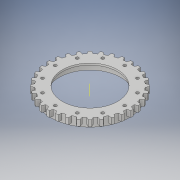
# Autodesk Inventor part: tableGear
Saved by Autodesk Inventor 2018 (Build 220112000, 112)
## iProperties
Created: 2018-04-17
Part Number: tableGear
Material: Generic
Document SubType Name: Modeling
Designer: Cole Tucker
Density: 1 g/cm^3
Appearance: Default
Author: Cole Tucker
Autodesk Inventor part; units mm, degrees
ref_plane "YZ Plane" through (0, 0, 0) normal (1, 0, 0) x (0, 1, 0)
ref_plane "XZ Plane" through (0, 0, 0) normal (0, 1, 0) x (-1, 0, 0)
ref_plane "XY Plane" through (0, 0, 0) normal (0, 0, 1) x (1, 0, 0)
sketch "Sketch1" plane through (0, 0, 0) normal (0, 1, 0) x (-1, 0, 0)
  circle A0 centre (0, 0) radius 29.21
  circle A1 centre (0, 0) radius 41.275
  dimension "d0" = 58.42
  dimension "d1" = 82.55
  constraints: 2 centre point, 2 coincident
  measures "d0" diameter of A0
  measures "d1" diameter of A1
extrude "Extrusion1" add sketch "Sketch1" along normal blind 8.89
sketch "Sketch2" plane through (0, 8.89, 0) normal (0, 1, 0) x (1, 0, 0)
  circle A0 centre (0, 0) radius 29.21 projected
  circle A1 centre (0, 0) radius 41.275 projected
  circle A2 centre (0, 0) radius 41.275 projected
  line L0 (-41.275, 0) -> (-44.45, 0)
  line L1 (-44.45, 0) -> (-44.45, 1.27)
  line L2 (-41.275, 0) -> (-40.5721, 0)
  line L3 (-40.5721, 0) -> (-40.5721, 2.54)
  line L4 (-40.5721, 2.54) -> (-44.45, 1.27)
  line L5 (-40.5721, 0) -> (-40.5721, -2.54)
  line L6 (-44.45, 0) -> (-44.45, -1.27)
  line L7 (-44.45, -1.27) -> (-40.5721, -2.54)
  dimension "d4" = 3.175
  dimension "d5" = 1.27
  dimension "d6" = 2.54
  dimension "d7" = 2.54
  dimension "d8" = 1.27
  constraints: 16 end point, 2 horizontal, 2 perpendicular, 1 horizontal alignment, 1 point on line, 1 vertical, 1 other
  measures "d4" distance of L0.start L0.end
  measures "d5" distance of L0.end L1.end
  measures "d6" distance of L2.end L3.end
  measures "d7" distance of L2.end L5.end
  measures "d8" distance of L0.end L6.end
extrude "Extrusion2" add sketch "Sketch2" against normal blind 6.35 contours L4 L3 L2 A1 | A1 L0 L1 L4 | L7 L6 L0 A1 | A1 L2 L5 L7
pattern_circular "Circular Pattern1" count 32 over 360 about axis through (0, 0, 0) along (0, 1, 0) of "Extrusion2"
sketch "Sketch3" plane through (0, 8.89, 0) normal (0, 1, 0) x (1, 0, 0)
  line L0 (-1.27, 44.45) -> (1.27, 44.45) projected
  line L1 (0, 44.45) -> (0, 29.21)
  circle A0 centre (0, 0) radius 29.21 projected
  point P0 (0, 36.752)
  constraints: 2 end point, 1 midpoint, 1 point on line, 1 vertical, 1 vertical alignment, 1 other
hole "Hole1" at (0, 8.89, -36.752) direction (0, -1, 0) diameter 3.175 end through all
pattern_circular "Circular Pattern2" count 12 over 360 about axis through (0, 0, 0) along (0, 1, 0) of "Hole1"
sketch "Sketch4" plane through (0, 0, 0) normal (0, -1, 0) x (1, 0, 0)
  circle A0 centre (0, 0) radius 32.71
  dimension "d24" = 65.42
  constraints: 1 centre point, 1 coincident
  measures "d24" diameter of A0
extrude "Extrusion3" cut sketch "Sketch4" against normal blind 7
body "Solid1"
